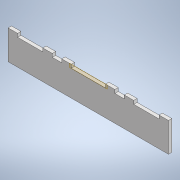
# Autodesk Inventor part: new_side_bottom
Saved by Autodesk Inventor 2020 (Build 240168000, 168)
## iProperties
Created: 2020-01-10
Part Number: new_side_bottom
Material: Generic
Document SubType Name: Modeling
Designer: erwin
Density: 1 g/cm^3
Appearance: Default
Author: erwin
Autodesk Inventor part; units mm, degrees
ref_plane "YZ Plane" through (0, 0, 0) normal (1, 0, 0) x (0, 1, 0)
ref_plane "XZ Plane" through (0, 0, 0) normal (0, 1, 0) x (-1, 0, 0)
ref_plane "XY Plane" through (0, 0, 0) normal (0, 0, 1) x (1, 0, 0)
ref_plane "Work Plane1" through (0, 0, 0) normal (0, 0, 1) x (1, 0, 0)
sketch "Sketch1" plane through (0, 0, 0) normal (0, 0, 1) x (1, 0, 0)
  line L0 (106.8, 0) -> (106.8, 3.6) projected
  line L1 (70.4, 3.6) -> (106.8, 3.6) projected
  line L2 (70.4, 3.6) -> (70.4, 0) projected
  line L3 (70.4, 0) -> (106.8, 0) projected
  line L4 (60.4, 0) -> (60.4, 3.6) projected
  line L5 (50.4, 3.6) -> (60.4, 3.6) projected
  line L6 (50.4, 3.6) -> (50.4, 0) projected
  line L7 (50.4, 0) -> (60.4, 0) projected
  line L8 (13.6, 3.6) -> (13.6, 0) projected
  line L9 (13.6, 0) -> (40.4, 0) projected
  line L10 (40.4, 0) -> (40.4, 3.6) projected
  line L11 (13.6, 3.6) -> (40.4, 3.6) projected
  line L12 (116.8, 3.6) -> (116.8, 0) projected
  line L13 (116.8, 0) -> (126.8, 0) projected
  line L14 (126.8, 0) -> (126.8, 3.6) projected
  line L15 (116.8, 3.6) -> (126.8, 3.6) projected
  line L16 (136.8, 3.6) -> (136.8, 0) projected
  line L17 (136.8, 0) -> (163.6, 0) projected
  line L18 (163.6, 0) -> (163.6, 3.6) projected
  line L19 (136.8, 3.6) -> (163.6, 3.6) projected
  line L20 (69.4, -27.6) -> (2.8, -27.6) projected
  line L21 (3.6, 0.6) -> (3.6, -27) projected
  line L22 (3.6, -30) -> (3.6, -27) projected
  line L23 (3.6, 0.6) -> (3.6, 3.6) projected
  line L24 (173.6, 0.6) -> (173.6, -27) projected
  line L25 (174.4, -27.45) -> (71.4, -27.45) projected
  line L26 (3.6, 3.6) -> (173.6, 3.6)
  line L27 (173.6, 3.6) -> (173.6, -27.45)
  line L28 (173.6, -27.45) -> (3.6, -27.45)
  line L29 (3.6, -27.45) -> (3.6, 3.6)
  point P0 (0, 0)
  point P1 (3.6, -27.45)
  constraints: 8 end point, 2 parallel, 1 horizontal, 1 perpendicular, 1 point on line
extrude "Extrusion1" add sketch "Sketch1" against normal blind 3.6 contours L0 L26 L12 L13 L14 L16 L17 L18 L27 L24 L25 L28 L22 L21 L23 L8 L9 L10 L6 L7 L4 L2 L3
sketch "Sketch2" plane through (3.6, -27.45, 0) normal (-1, 0, 0) x (0, 0, 1)
  line L0 (0, 5.45) -> (-3.6, 5.45) projected
  line L1 (-3.6, 5.45) -> (-3.6, 10.45) projected
  line L2 (-3.6, 10.45) -> (0, 10.45) projected
  line L3 (0, 10.45) -> (0, 5.45) projected
  line L4 (0, 20.45) -> (-3.6, 20.45) projected
  line L5 (-3.6, 20.45) -> (-3.6, 25.45) projected
  line L6 (-3.6, 25.45) -> (0, 25.45) projected
  line L7 (0, 25.45) -> (0, 20.45) projected
  point P0 (0, 27.45)
extrude "Extrusion2" add sketch "Sketch2" along normal blind 3.6
sketch "Sketch3" plane through (0, 0, 0) normal (0, 0, 1) x (1, 0, 0)
  line L0 (60.4, 3.6) -> (60.4, 0) projected
  line L1 (60.4, 0) -> (50.4, 0) projected
  line L2 (50.4, 0) -> (50.4, 3.6) projected
  line L3 (50.4, 3.6) -> (40.4, 3.6) projected
  line L4 (40.4, 3.6) -> (40.4, 0) projected
  line L5 (40.4, 0) -> (13.6, 0) projected
  line L6 (13.6, 0) -> (13.6, 3.6) projected
  line L7 (13.6, 3.6) -> (3.6, 3.6) projected
  line L8 (3.6, 3.6) -> (3.6, -2) projected
  line L9 (3.6, -2) -> (0, -2) projected
  line L10 (0, -7) -> (0, -2) projected
  line L11 (3.6, -7) -> (0, -7) projected
  line L12 (3.6, -7) -> (3.6, -17) projected
  line L13 (3.6, -17) -> (0, -17) projected
  line L14 (0, -22) -> (0, -17) projected
  line L15 (3.6, -22) -> (0, -22) projected
  line L16 (3.6, -22) -> (3.6, -27.45) projected
  line L17 (3.6, -27.45) -> (173.6, -27.45) projected
  line L18 (173.6, -27.45) -> (173.6, 3.6) projected
  line L19 (173.6, 3.6) -> (163.6, 3.6) projected
  line L20 (163.6, 3.6) -> (163.6, 0) projected
  line L21 (163.6, 0) -> (136.8, 0) projected
  line L22 (136.8, 0) -> (136.8, 3.6) projected
  line L23 (136.8, 3.6) -> (126.8, 3.6) projected
  line L24 (126.8, 3.6) -> (126.8, 0) projected
  line L25 (126.8, 0) -> (116.8, 0) projected
  line L26 (116.8, 0) -> (116.8, 3.6) projected
  line L27 (116.8, 3.6) -> (106.8, 3.6) projected
  line L28 (106.8, 3.6) -> (106.8, 0) projected
  line L29 (106.8, 0) -> (70.4, 0) projected
  line L30 (70.4, 0) -> (70.4, 3.6) projected
  line L31 (70.4, 3.6) -> (60.4, 3.6) projected
  line L32 (16.6, -13.5) -> (-9.4, -13.5)
  line L33 (-9.4, -13.5) -> (-9.4, -10.5)
  line L34 (-9.4, -10.5) -> (16.6, -10.5)
  line L35 (16.6, -10.5) -> (16.6, -13.5)
  line L36 (3.6, -7) -> (3.6, -17) projected
  line L37 (16.6, -13.5) -> (-9.4, -10.5) construction
  line L38 (-9.4, -13.5) -> (16.6, -10.5) construction
  line L39 (10.6, -16) -> (7.6, -16)
  line L40 (7.6, -16) -> (7.6, -8)
  line L41 (7.6, -8) -> (10.6, -8)
  line L42 (10.6, -8) -> (10.6, -16)
  line L43 (10.6, -16) -> (7.6, -8) construction
  line L44 (7.6, -16) -> (10.6, -8) construction
  line L45 (16.6, -12) -> (-9.4, -12) construction
  point P0 (0, 0)
  point P1 (3.6, -12)
  point P2 (9.1, -12)
  point P3 (9.1, -12)
  point P4 (7.6, -13.5)
  point P5 (10.6, -13.5)
  point P6 (10.6, -10.5)
  point P7 (7.6, -10.5)
  dimension "d4" = 26
  dimension "d5" = 3
  dimension "d6" = 3
  dimension "d7" = 8
  dimension "d8" = 4
  constraints: 26 end point, 8 midpoint, 4 parallel, 2 horizontal, 2 perpendicular, 1 point on line
  measures "d4" distance of L32.start L32.end
  measures "d5" distance of L32.end L33.end
  measures "d6" distance of L39.start L39.end
  measures "d7" distance between parallel lines of L41 L39
  measures "d8" distance between parallel lines of L12 L40
extrude "Extrusion3" cut sketch "Sketch3" against normal through all contours L34 L40 L32 L12 | L12 L32 L33 L34 | L40 L41 L42 L34 | L34 L42 L32 L40 | L32 L42 L39 L40 | L34 L35 L32 L42
ref_plane "Work Plane2" through (88.6, 0, 0) normal (-1, 0, 0) x (0, 0, 1)
sketch "Sketch4" plane through (0, 0, 0) normal (0, 0, 1) x (1, 0, 0)
  line L0 (3.6, -10.5) -> (7.6, -10.5) projected
  line L1 (7.6, -10.5) -> (7.6, -8) projected
  line L2 (7.6, -8) -> (10.6, -8) projected
  line L3 (10.6, -8) -> (10.6, -10.5) projected
  line L4 (10.6, -10.5) -> (16.6, -10.5) projected
  line L5 (16.6, -10.5) -> (16.6, -13.5) projected
  line L6 (16.6, -13.5) -> (10.6, -13.5) projected
  line L7 (10.6, -13.5) -> (10.6, -16) projected
  line L8 (10.6, -16) -> (7.6, -16) projected
  line L9 (7.6, -16) -> (7.6, -13.5) projected
  line L10 (7.6, -13.5) -> (3.6, -13.5) projected
  line L11 (3.6, -13.5) -> (3.6, -17) projected
  line L12 (3.6, -17) -> (0, -17) projected
  line L13 (0, -22) -> (0, -17) projected
  line L14 (3.6, -22) -> (0, -22) projected
  line L15 (3.6, -22) -> (3.6, -27.45) projected
  line L16 (3.6, -27.45) -> (173.6, -27.45) projected
  line L17 (173.6, -27.45) -> (173.6, 3.6) projected
  line L18 (173.6, 3.6) -> (163.6, 3.6) projected
  line L19 (163.6, 3.6) -> (163.6, 0) projected
  line L20 (163.6, 0) -> (136.8, 0) projected
  line L21 (136.8, 0) -> (136.8, 3.6) projected
  line L22 (136.8, 3.6) -> (126.8, 3.6) projected
  line L23 (126.8, 3.6) -> (126.8, 0) projected
  line L24 (126.8, 0) -> (116.8, 0) projected
  line L25 (116.8, 0) -> (116.8, 3.6) projected
  line L26 (116.8, 3.6) -> (106.8, 3.6) projected
  line L27 (106.8, 3.6) -> (106.8, 0) projected
  line L28 (106.8, 0) -> (70.4, 0) projected
  line L29 (70.4, 0) -> (70.4, 3.6) projected
  line L30 (70.4, 3.6) -> (60.4, 3.6) projected
  line L31 (60.4, 3.6) -> (60.4, 0) projected
  line L32 (60.4, 0) -> (50.4, 0) projected
  line L33 (50.4, 0) -> (50.4, 3.6) projected
  line L34 (50.4, 3.6) -> (40.4, 3.6) projected
  line L35 (40.4, 3.6) -> (40.4, 0) projected
  line L36 (40.4, 0) -> (13.6, 0) projected
  line L37 (13.6, 0) -> (13.6, 3.6) projected
  line L38 (13.6, 3.6) -> (3.6, 3.6) projected
  line L39 (3.6, 3.6) -> (3.6, -2) projected
  line L40 (3.6, -2) -> (0, -2) projected
  line L41 (0, -7) -> (0, -2) projected
  line L42 (3.6, -7) -> (0, -7) projected
  line L43 (3.6, -7) -> (3.6, -10.5) projected
  circle A0 centre (2.6101, -16.0101) radius 1.4
  line L44 (3.6, -17) -> (1.6201, -17) construction
  line L45 (1.6201, -17) -> (1.6201, -15.0201) construction
  line L46 (1.6201, -15.0201) -> (3.6, -15.0201) construction
  line L47 (3.6, -15.0201) -> (3.6, -17) construction
  line L48 (3.6, -17) -> (1.6201, -15.0201) construction
  line L49 (1.6201, -17) -> (3.6, -15.0201) construction
  circle A1 centre (14.5899, 0.9899) radius 1.4
  line L50 (15.5799, 0) -> (13.6, 0) construction
  line L51 (13.6, 0) -> (13.6, 1.9799) construction
  line L52 (13.6, 1.9799) -> (15.5799, 1.9799) construction
  line L53 (15.5799, 1.9799) -> (15.5799, 0) construction
  line L54 (15.5799, 0) -> (13.6, 1.9799) construction
  line L55 (13.6, 0) -> (15.5799, 1.9799) construction
  circle A2 centre (59.4101, 0.9899) radius 1.4
  line L56 (60.4, 0) -> (58.4201, 0) construction
  line L57 (58.4201, 0) -> (58.4201, 1.9799) construction
  line L58 (58.4201, 1.9799) -> (60.4, 1.9799) construction
  line L59 (60.4, 1.9799) -> (60.4, 0) construction
  line L60 (60.4, 0) -> (58.4201, 1.9799) construction
  line L61 (58.4201, 0) -> (60.4, 1.9799) construction
  circle A3 centre (51.3899, 0.9899) radius 1.4
  line L62 (52.3799, 0) -> (50.4, 0) construction
  line L63 (50.4, 0) -> (50.4, 1.9799) construction
  line L64 (50.4, 1.9799) -> (52.3799, 1.9799) construction
  line L65 (52.3799, 1.9799) -> (52.3799, 0) construction
  line L66 (52.3799, 0) -> (50.4, 1.9799) construction
  line L67 (50.4, 0) -> (52.3799, 1.9799) construction
  circle A4 centre (39.4101, 0.9899) radius 1.4
  line L68 (40.4, 0) -> (38.4201, 0) construction
  line L69 (38.4201, 0) -> (38.4201, 1.9799) construction
  line L70 (38.4201, 1.9799) -> (40.4, 1.9799) construction
  line L71 (40.4, 1.9799) -> (40.4, 0) construction
  line L72 (40.4, 0) -> (38.4201, 1.9799) construction
  line L73 (38.4201, 0) -> (40.4, 1.9799) construction
  circle A5 centre (71.3899, 0.9899) radius 1.4
  line L74 (72.3799, 0) -> (70.4, 0) construction
  line L75 (70.4, 0) -> (70.4, 1.9799) construction
  line L76 (70.4, 1.9799) -> (72.3799, 1.9799) construction
  line L77 (72.3799, 1.9799) -> (72.3799, 0) construction
  line L78 (72.3799, 0) -> (70.4, 1.9799) construction
  line L79 (70.4, 0) -> (72.3799, 1.9799) construction
  circle A6 centre (2.6101, -1.0101) radius 1.4
  line L80 (3.6, -2) -> (1.6201, -2) construction
  line L81 (1.6201, -2) -> (1.6201, -0.0201) construction
  line L82 (1.6201, -0.0201) -> (3.6, -0.0201) construction
  line L83 (3.6, -0.0201) -> (3.6, -2) construction
  line L84 (3.6, -2) -> (1.6201, -0.0201) construction
  line L85 (1.6201, -2) -> (3.6, -0.0201) construction
  circle A7 centre (2.6101, -7.9899) radius 1.4
  line L86 (3.6, -8.9799) -> (1.6201, -8.9799) construction
  line L87 (1.6201, -8.9799) -> (1.6201, -7) construction
  line L88 (1.6201, -7) -> (3.6, -7) construction
  line L89 (3.6, -7) -> (3.6, -8.9799) construction
  line L90 (3.6, -8.9799) -> (1.6201, -7) construction
  line L91 (1.6201, -8.9799) -> (3.6, -7) construction
  circle A8 centre (2.6101, -22.9899) radius 1.4
  line L92 (3.6, -23.9799) -> (1.6201, -23.9799) construction
  line L93 (1.6201, -23.9799) -> (1.6201, -22) construction
  line L94 (1.6201, -22) -> (3.6, -22) construction
  line L95 (3.6, -22) -> (3.6, -23.9799) construction
  line L96 (3.6, -23.9799) -> (1.6201, -22) construction
  line L97 (1.6201, -23.9799) -> (3.6, -22) construction
  point P0 (0, 0)
  dimension "d11" = 2.8
  dimension "d12" = 2.8
  dimension "d14" = 2.8
  dimension "d16" = 2.8
  dimension "d18" = 2.8
  dimension "d20" = 2.8
  dimension "d22" = 2.8
  dimension "d24" = 2.8
  dimension "d26" = 2.8
  constraints: 108 end point, 18 midpoint, 18 parallel, 18 perpendicular, 9 horizontal, 27 other
extrude "Extrusion4" cut sketch "Sketch4" against normal through all contours A7 L42 L43 | L43 A7 | L42 A7 | A6 L39 L40 | L40 A6 | L39 A6 | A1 L36 L37 | L37 A1 | L36 A1 | A0 L11 | L11 L12 A0 | A4 L35 L36 | L36 A4 | A0 L12 | L35 A4 | A8 L14 | L14 L15 A8 | A3 L32 L33 | L33 A3 | A8 L15 | L32 A3 | A2 L31 L32 | L32 A2 | L31 A2 | A5 L28 L29 | L29 A5 | L28 A5
mirror "Mirror1" about plane through (88.6, 0, 0) normal (-1, 0, 0) of "Extrusion4", "Extrusion3", "Extrusion2"
move faces "Move1" translate (0, -2.55, 0) faces at (60.2667, -27.45, -1.2)
sketch "Sketch5" plane through (0, -27.45, 0) normal (-1, 0, 0) x (0, 0, 1)
  line L0 (-1.8, -0.15) -> (-1.8, 3.45) projected
  line L1 (-1.8, -0.15) -> (-5.1628, -0.15)
  line L2 (-5.1628, -0.15) -> (-5.1628, 3.45)
  line L3 (-5.1628, 3.45) -> (-1.8, 3.45)
  line L4 (-1.8, 3.45) -> (-1.8, -0.15)
  point P0 (0, 27.45)
  point P1 (-1.8, 3.45)
  constraints: 8 end point, 2 parallel, 1 horizontal, 1 perpendicular
extrude "Extrusion5" cut sketch "Sketch5" against normal through all
thicken "Thicken1" operation add thickness 0.4 both sides no extend neighbours yes toward (0, 1, 0) faces at (60.2667, -24, -3)
thicken "Thicken2" operation add thickness 0.4 both sides no extend neighbours yes toward (0, -1, 0) faces at (60.2667, -27.6, -3)
equation "\"d0\" = wood_thickness"
equation "\"d2\" = wood_thickness"
equation "\"d4\" = 2 * screw_depth"
equation "\"d5\" = screw_diameter"
equation "\"d6\" = screw_nut_thickness"
equation "\"d7\" = screw_nut_width"
equation "\"d11\" = bit_diameter"
equation "\"d12\" = d13"
equation "\"d14\" = d15"
equation "\"d16\" = d17"
equation "\"d18\" = d19"
equation "\"d20\" = d21"
equation "\"d22\" = d23"
equation "\"d24\" = d25"
equation "\"d26\" = d27"
equation "\"d35\" = rails_slack_extra"
equation "\"d36\" = 0.5 * rails_slack_extra"
equation "\"d37\" = rails_slack_extra"
equation "\"d38\" = 0.5 * rails_slack_extra"
equation "\"wood_thickness\" = 3.6"
equation "\"screw_depth\" = 13"
equation "\"screw_diameter\" = 3"
equation "\"screw_nut_thickness\" = 3"
equation "\"screw_nut_width\" = 8"
equation "\"bit_diameter\" = 2.8"
equation "\"d13\" = 2.8"
equation "\"d15\" = 2.8"
equation "\"d17\" = 2.8"
equation "\"d19\" = 2.8"
equation "\"d21\" = 2.8"
equation "\"d23\" = 2.8"
equation "\"d25\" = 2.8"
equation "\"d27\" = 2.8"
equation "\"rails_slack_extra\" = 0.4"
body "Solid1"
